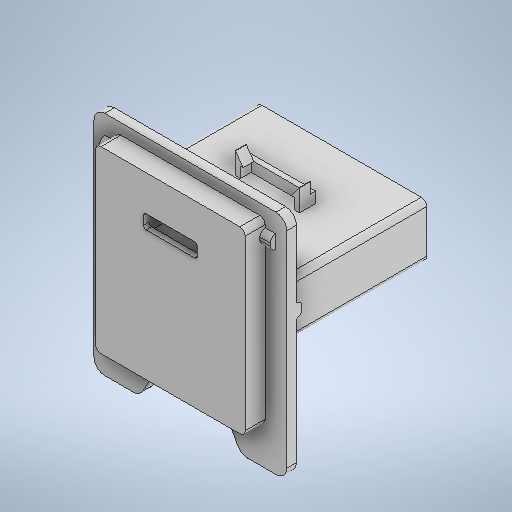
# Autodesk Inventor part: PS2 USB C PD Mount
Saved by Autodesk Inventor 2025 (Build 290162000, 162)
## iProperties
Created: 2024-07-11
Part Number: PS2 USB C PD Mount
Material: Generic
Document SubType Name: Modeling
Designer: chuca
Density: 1 g/cm^3
Appearance: Default
Author: chuca
Autodesk Inventor part; units mm, degrees
ref_plane "YZ Plane" through (0, 0, 0) normal (1, 0, 0) x (0, 1, 0)
ref_plane "XZ Plane" through (0, 0, 0) normal (0, 1, 0) x (-1, 0, 0)
ref_plane "XY Plane" through (0, 0, 0) normal (0, 0, 1) x (1, 0, 0)
sketch "Sketch1" plane through (0, 0, 0) normal (0, 0, 1) x (1, 0, 0)
  line L0 (17.9, -19.1) -> (17.9, 19.1)
  line L1 (15.9, 21.1) -> (-15.9, 21.1)
  line L2 (-17.9, 19.1) -> (-17.9, -19.1)
  line L3 (-15.9, -21.1) -> (-10.5924, -21.1)
  line L4 (17.9, -21.1) -> (-17.9, 21.1) construction
  line L5 (17.9, 21.1) -> (-17.9, -21.1) construction
  line L6 (-7.4, -17.4) -> (7.4, -17.4)
  line L7 (-7.4, -17.4) -> (-8.833, -20.051)
  line L8 (7.4, -17.4) -> (8.833, -20.051)
  line L9 (10.5924, -21.1) -> (15.9, -21.1)
  line L10 (-9.4, -21.1) -> (9.4, -21.1)
  arc A0 (-15.9, 21.1) -> (-17.9, 19.1) centre (-15.9, 19.1) ccw
  arc A1 (17.9, 19.1) -> (15.9, 21.1) centre (15.9, 19.1) ccw
  arc A2 (15.9, -21.1) -> (17.9, -19.1) centre (15.9, -19.1) ccw
  arc A3 (8.833, -20.051) -> (10.5924, -21.1) centre (10.5924, -19.1) ccw
  arc A4 (-10.5924, -21.1) -> (-8.833, -20.051) centre (-10.5924, -19.1) ccw
  arc A5 (-17.9, -19.1) -> (-15.9, -21.1) centre (-15.9, -19.1) ccw
  point P0 (0, 0)
  dimension "d0" = 35.8
  dimension "d1" = 42.2
  dimension "d2" = 38.5
  dimension "d3" = 10.5
  dimension "d4" = 10.5
  dimension "d5" = 8.5
  dimension "d6" = 8.5
  dimension "d7" = 2
  constraints: 22 end point, 12 point on circle, 12 point on line, 12 tangent, 6 centre point, 5 equal radius, 4 parallel, 2 midpoint, 1 horizontal, 1 perpendicular, 1 vertical
  measures "d0" distance of L5.start L4.end
  measures "d1" distance of L4.start L5.start
  measures "d2" distance between parallel lines of L1 L6
  measures "d3" distance from line of L2 L6.start
  measures "d4" distance from line of L0 L6.end
  measures "d5" distance from line of L2 L10.start
  measures "d6" distance of L4.start L10.end
  measures "d7" radius of A0
extrude "Extrusion1" add sketch "Sketch1" along normal blind 1.8
sketch "Sketch2" plane through (0, 0, 1.8) normal (0, 0, 1) x (1, 0, 0)
  line L0 (-15.85, 15.1) -> (15.85, 15.1)
  line L1 (15.85, 15.1) -> (15.85, 17.6)
  line L2 (15.85, 17.6) -> (-15.85, 17.6)
  line L3 (-15.85, 17.6) -> (-15.85, 15.1)
  line L4 (-15.85, 15.1) -> (15.85, 17.6) construction
  line L5 (15.85, 15.1) -> (-15.85, 17.6) construction
  line L6 (15.9, 21.1) -> (-15.9, 21.1) projected
  point P0 (0, 0)
  point P1 (0, 16.35)
  point P2 (0, 16.35)
  point P3 (15.85, 16.35)
  point P4 (-15.85, 16.35)
  dimension "d10" = 2.5
  dimension "d11" = 6
  dimension "d12" = 31.7
  constraints: 12 end point, 5 midpoint, 2 parallel, 1 horizontal, 1 perpendicular, 1 vertical alignment
  measures "d10" distance of L1.end L0.end
  measures "d11" distance between parallel lines of L6 L0
  measures "d12" distance of point (15.85, 16.35) point (-15.85, 16.35)
extrude "Extrusion2" add sketch "Sketch2" along normal blind 1
fillet "Fillet1" radius 1 2 edges at (0, 17.6, 2.8) (0, 15.1, 2.8)
sketch "Sketch3" plane through (0, 0, 1.8) normal (0, 0, 1) x (1, 0, 0)
  line L0 (-12.9, 19.1) -> (12.9, 19.1)
  line L1 (13.9, 18.1) -> (13.9, -13.2)
  line L2 (12.9, -14.2) -> (-12.9, -14.2)
  line L3 (-13.9, -13.2) -> (-13.9, 18.1)
  line L4 (15.9, 21.1) -> (-15.9, 21.1) projected
  line L5 (-13.9, 2.9131) -> (-17.9, 2.9131)
  line L6 (-17.9, 19.1) -> (-17.9, -19.1) projected
  line L7 (13.9, 2.9131) -> (17.9, 2.9131)
  line L8 (17.9, -19.1) -> (17.9, 19.1) projected
  arc A0 (-12.9, 19.1) -> (-13.9, 18.1) centre (-12.9, 18.1) ccw
  arc A1 (13.9, 18.1) -> (12.9, 19.1) centre (12.9, 18.1) ccw
  arc A2 (12.9, -14.2) -> (13.9, -13.2) centre (12.9, -13.2) ccw
  arc A3 (-13.9, -13.2) -> (-12.9, -14.2) centre (-12.9, -13.2) ccw
  point P0 (0, 0)
  point P1 (13.9, -14.2)
  point P2 (13.9, 19.1)
  point P3 (-13.9, -14.2)
  dimension "d16" = 27.8
  dimension "d17" = 33.3
  dimension "d18" = 2
  dimension "d19" = 1
  constraints: 12 end point, 12 point on line, 8 point on circle, 8 tangent, 4 centre point, 3 equal radius, 2 horizontal, 2 parallel, 1 collinear, 1 perpendicular
  measures "d16" distance of point (13.9, -14.2) point (-13.9, -14.2)
  measures "d17" distance of point (13.9, 19.1) point (13.9, -14.2)
  measures "d18" distance between parallel lines of L4 L0
  measures "d19" radius of A0
extrude "Extrusion3" add sketch "Sketch3" along normal blind 3.7
sketch "Sketch4" plane through (0, 0, 0) normal (0, 0, -1) x (-1, 0, 0)
  line L0 (-17.9, -19.1) -> (-17.9, 19.1) projected
  line L1 (17.9, 19.1) -> (17.9, -19.1) projected
  line L2 (-17.9, 6.6) -> (17.9, 6.6)
  line L3 (17.9, 6.6) -> (17.9, 4.1)
  line L4 (17.9, 4.1) -> (-17.9, 4.1)
  line L5 (-17.9, 4.1) -> (-17.9, 6.6)
  line L6 (-15.9, 21.1) -> (15.9, 21.1) projected
  point P0 (0, 0)
  dimension "d22" = 2.5
  dimension "d23" = 17
  constraints: 8 end point, 2 parallel, 2 point on line, 1 horizontal, 1 perpendicular
  measures "d22" distance between parallel lines of L4 L2
  measures "d23" distance between parallel lines of L6 L4
extrude "Extrusion4" add sketch "Sketch4" along normal blind 1
fillet "Fillet2" radius 1 2 edges at (0, 6.6, -1) (0, 4.1, -1)
sketch "Sketch5" plane through (0, 0, 0) normal (0, 0, -1) x (-1, 0, 0)
  line L0 (-14.8, 8.9) -> (14.8, 8.9)
  line L1 (15.8, 7.9) -> (15.8, -0.1)
  line L2 (14.8, -1.1) -> (-14.8, -1.1)
  line L3 (-15.8, -0.1) -> (-15.8, 7.9)
  line L4 (-15.9, 21.1) -> (15.9, 21.1) projected
  line L5 (-17.9, 6.6) -> (-17.9, 19.1) projected
  line L6 (17.9, 4.1) -> (17.9, -19.1) projected
  arc A0 (-15.8, -0.1) -> (-14.8, -1.1) centre (-14.8, -0.1) ccw
  arc A1 (-14.8, 8.9) -> (-15.8, 7.9) centre (-14.8, 7.9) ccw
  arc A2 (15.8, 7.9) -> (14.8, 8.9) centre (14.8, 7.9) ccw
  arc A3 (14.8, -1.1) -> (15.8, -0.1) centre (14.8, -0.1) ccw
  point P0 (0, 0)
  point P1 (0, 8.9)
  dimension "d27" = 22.2
  dimension "d28" = 2.1
  dimension "d29" = 10
  dimension "d30" = 2.1
  dimension "d31" = 1
  constraints: 8 end point, 8 point on circle, 8 tangent, 4 centre point, 3 equal radius, 2 parallel, 1 horizontal, 1 midpoint, 1 perpendicular
  measures "d27" distance between parallel lines of L4 L2
  measures "d28" distance between parallel lines of L5 L3
  measures "d29" distance from line of point (0, 8.9) L2
  measures "d30" distance between parallel lines of L6 L1
  measures "d31" radius of A0
extrude "Extrusion5" add sketch "Sketch5" along normal blind 26.3
sketch "Sketch6" plane through (0, 0, 0) normal (0, 0, -1) x (-1, 0, 0)
  line L0 (-5, 16.9799) -> (5, 16.9799)
  line L1 (5, 16.9799) -> (5, 8.9)
  line L2 (5, 8.9) -> (-5, 8.9)
  line L3 (-5, 8.9) -> (-5, 16.9799)
  line L4 (14.8, 8.9) -> (-14.8, 8.9) projected
  line L5 (5, 16.9799) -> (17.9, 16.9799)
  line L6 (17.9, 19.1) -> (17.9, 6.6) projected
  line L7 (-5, 16.9799) -> (-17.9, 16.9799)
  line L8 (-17.9, -19.1) -> (-17.9, 19.1) projected
  point P0 (0, 0)
  point P1 (-5, 12.94)
  dimension "d34" = 10
  constraints: 12 end point, 4 point on line, 2 horizontal, 2 parallel, 1 collinear, 1 midpoint, 1 perpendicular
  measures "d34" distance from line of point (-5, 12.94) L1
extrude "Extrusion6" cut sketch "Sketch6" against normal blind 4.5
sketch "Sketch7" plane through (-14.8, 8.9, -26.3) normal (0, 1, 0) x (1, 0, 0)
  line L0 (9.8, -30.8) -> (19.8, -30.8) projected
  line L1 (14.8, -30.8) -> (14.8, -11.8)
  line L2 (8.8, -11.8) -> (20.8, -11.8)
  line L3 (20.8, -11.8) -> (20.8, -10.8)
  line L4 (20.8, -10.8) -> (8.8, -10.8)
  line L5 (8.8, -10.8) -> (8.8, -11.8)
  line L6 (20.8, -11.8) -> (20.8, -13.8)
  line L7 (20.8, -13.8) -> (19.8, -13.8)
  line L8 (19.8, -13.8) -> (19.8, -11.8)
  line L9 (8.8, -11.8) -> (8.8, -13.8)
  line L10 (8.8, -13.8) -> (9.8, -13.8)
  line L11 (9.8, -13.8) -> (9.8, -11.8)
  point P0 (14.8, -26.3)
  dimension "d37" = 19
  dimension "d38" = 12
  dimension "d39" = 1
  dimension "d40" = 1
  dimension "d41" = 2
  constraints: 22 end point, 5 perpendicular, 3 vertical, 2 equal length, 2 midpoint, 2 parallel, 2 point on line, 1 horizontal
  measures "d37" distance of L1.end L1.start
  measures "d38" distance of L3.end L4.end
  measures "d39" distance of L2.end L3.end
  measures "d40" distance between parallel lines of L8 L6
  measures "d41" distance between parallel lines of L2 L7
extrude "Extrusion7" add sketch "Sketch7" along normal blind 2
sketch "Sketch8" plane through (-14.8, 10.9, -26.3) normal (0, 1, 0) x (1, 0, 0)
  line L0 (9.8, -11.8) -> (19.8, -11.8) projected
  line L1 (20.8, -13.8) -> (20.8, -10.8) projected
  line L2 (19.8, -11.8) -> (20.8, -11.8)
  line L3 (20.8, -11.8) -> (20.8, -13.8)
  line L4 (20.8, -13.8) -> (19.8, -13.8)
  line L5 (19.8, -13.8) -> (19.8, -11.8)
  line L6 (9.8, -11.8) -> (9.8, -13.8) projected
  line L7 (8.8, -13.8) -> (8.8, -10.8) projected
  line L8 (9.8, -11.8) -> (8.8, -11.8)
  line L9 (8.8, -11.8) -> (8.8, -13.8)
  line L10 (8.8, -13.8) -> (9.8, -13.8)
  line L11 (9.8, -13.8) -> (9.8, -11.8)
  point P0 (14.8, -26.3)
  constraints: 16 end point, 4 parallel, 2 horizontal, 2 perpendicular
extrude "Extrusion8" add sketch "Sketch8" along normal blind 2
sketch "Sketch9" plane through (5, 8.9, -14.5) normal (-1, 0, 0) x (0, 0, 1)
  line L0 (0, 2) -> (0, 4) projected
  line L1 (2, 0) -> (2, 4) projected
  line L2 (0, 4) -> (2, 4)
  line L3 (2, 4) -> (2, 2)
  line L4 (2, 2) -> (0, 2)
  line L5 (0, 2) -> (0, 4)
  point P0 (14.5, -8.9)
  constraints: 8 end point, 2 parallel, 1 horizontal, 1 midpoint, 1 perpendicular
extrude "Extrusion9" add sketch "Sketch9" along normal blind 0.5
chamfer "Chamfer1" distance 2 angle 35 1 edges at (4.5, 12.9, -13.5) measured on face at (4.5, 11.5667, -13.8333)
mirror "Mirror1" about plane through (0, 0, 0) normal (1, 0, 0) of "Extrusion9", "Chamfer1"
sketch "Sketch10" plane through (0, 0, 4.5) normal (0, 0, -1) x (-1, 0, 0)
  line L0 (-4.5, 9.9) -> (4.5, 9.9)
  line L1 (5, 10.4) -> (5, 12)
  line L2 (4.5, 12.5) -> (-4.5, 12.5)
  line L3 (-5, 12) -> (-5, 10.4)
  line L4 (5, 8.9) -> (-5, 8.9) projected
  line L5 (-5, 8.9) -> (-5, 16.9799) projected
  arc A0 (-5, 10.4) -> (-4.5, 9.9) centre (-4.5, 10.4) ccw
  arc A1 (-4.5, 12.5) -> (-5, 12) centre (-4.5, 12) ccw
  arc A2 (5, 12) -> (4.5, 12.5) centre (4.5, 12) ccw
  arc A3 (4.5, 9.9) -> (5, 10.4) centre (4.5, 10.4) ccw
  point P0 (0, 0)
  point P1 (-5, 11.2)
  dimension "d51" = 1
  dimension "d52" = 10
  dimension "d53" = 0.5
  dimension "d54" = 2.6
  constraints: 8 end point, 8 point on circle, 8 tangent, 4 centre point, 3 equal radius, 2 parallel, 1 horizontal, 1 midpoint, 1 perpendicular, 1 point on line
  measures "d51" distance between parallel lines of L4 L0
  measures "d52" distance from line of point (-5, 11.2) L1
  measures "d53" radius of A0
  measures "d54" distance between parallel lines of L0 L2
extrude "Extrusion10" cut sketch "Sketch10" against normal blind 2
body "Solid1"
